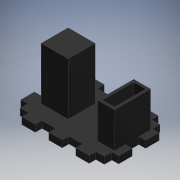
# Autodesk Inventor part: top
Saved by Autodesk Inventor 2019 (Build 230136000, 136)
## iProperties
Created: 2018-06-06
Part Number: top
Material: PBT Plastic Black
Document SubType Name: Modeling
Designer: stra92745
Density: 1.31 g/cm^3
Appearance: Smooth - White
Author: stra92745
Autodesk Inventor part; units mm, degrees
ref_plane "YZ Plane" through (0, 0, 0) normal (1, 0, 0) x (0, 1, 0)
ref_plane "XZ Plane" through (0, 0, 0) normal (0, 1, 0) x (-1, 0, 0)
ref_plane "XY Plane" through (0, 0, 0) normal (0, 0, 1) x (1, 0, 0)
sketch "Sketch1" plane through (0, 0, 0) normal (0, 1, 0) x (-1, 0, 0)
  line L0 (0, 0) -> (-58, 0)
  line L1 (-58, 0) -> (-58, -41)
  line L2 (-58, -41) -> (0, -41)
  line L3 (0, -41) -> (0, 0)
  line L4 (-45.5, -30) -> (-52.5, -30)
  line L5 (-52.5, -30) -> (-52.5, -11.5)
  line L6 (-52.5, -11.5) -> (-45.5, -11.5)
  line L7 (-45.5, -11.5) -> (-45.5, -30)
  dimension "d0" = 58
  dimension "d1" = 41
  dimension "d2" = 11.5
  dimension "d3" = 11
  dimension "d4" = 7
  dimension "d5" = 5.5
  constraints: 16 end point, 4 parallel, 2 horizontal, 2 perpendicular
  measures "d0" distance of L2.end L1.end
  measures "d1" distance of L1.end L0.end
  measures "d2" distance between parallel lines of L0 L6
  measures "d3" distance between parallel lines of L2 L4
  measures "d4" distance of L5.end L6.end
  measures "d5" distance between parallel lines of L1 L5
extrude "Extrusion1" add sketch "Sketch1" along normal blind 4
sketch "Sketch2" plane through (0, 4, 0) normal (0, 1, 0) x (1, 0, 0)
  line L0 (45.5, 11.5) -> (45.5, 30) projected
  line L1 (45.5, 30) -> (52.5, 30) projected
  line L2 (52.5, 30) -> (52.5, 11.5) projected
  line L3 (52.5, 11.5) -> (45.5, 11.5) projected
  line L4 (54, 31.5) -> (44, 31.5)
  line L5 (44, 31.5) -> (44, 10)
  line L6 (44, 10) -> (54, 10)
  line L7 (54, 10) -> (54, 31.5)
  point P0 (0, 0)
  dimension "d8" = 1.5
  constraints: 8 end point, 3 other
  measures "d8" distance between parallel lines of L1 L4
extrude "Extrusion2" add sketch "Sketch2" along normal blind 21
sketch "Sketch3" plane through (0, 4, 0) normal (0, 1, 0) x (1, 0, 0)
  line L0 (58, 41) -> (0, 41) construction
  line L1 (0, 41) -> (0, 0) construction
  line L2 (0, 0) -> (58, 0) construction
  line L3 (58, 0) -> (58, 41) construction
  line L4 (4, 37) -> (54, 37) construction
  line L5 (54, 37) -> (54, 4) construction
  line L6 (54, 4) -> (4, 4) construction
  line L7 (4, 4) -> (4, 37) construction
  line L8 (0, 20.5) -> (58, 20.5) construction
  line L9 (29, 0) -> (29, 41) construction
  line L10 (0, 16.5) -> (4, 16.5)
  line L11 (4, 16.5) -> (4, 20.5)
  line L12 (0, 16.5) -> (0, 20.5)
  line L13 (0, 8.5) -> (4, 8.5)
  line L14 (4, 8.5) -> (4, 4)
  line L15 (4, 4) -> (9, 4)
  line L16 (9, 4) -> (9, 0)
  line L17 (9, 0) -> (0, 0)
  line L18 (0, 0) -> (0, 8.5)
  line L19 (17, 4) -> (17, 0)
  line L20 (17, 0) -> (25, 0)
  line L21 (25, 0) -> (25, 4)
  line L22 (25, 4) -> (17, 4)
  line L23 (0, 24.5) -> (4, 24.5)
  line L24 (4, 24.5) -> (4, 20.5)
  line L25 (0, 24.5) -> (0, 20.5)
  line L26 (0, 32.5) -> (4, 32.5)
  line L27 (4, 32.5) -> (4, 37)
  line L28 (4, 37) -> (9, 37)
  line L29 (9, 37) -> (9, 41)
  line L30 (9, 41) -> (0, 41)
  line L31 (0, 41) -> (0, 32.5)
  line L32 (17, 37) -> (17, 41)
  line L33 (17, 41) -> (25, 41)
  line L34 (25, 41) -> (25, 37)
  line L35 (25, 37) -> (17, 37)
  line L36 (58, 41) -> (58, 0) construction
  line L37 (54, 4) -> (54, 37) construction
  line L38 (58, 16.5) -> (54, 16.5)
  line L39 (54, 16.5) -> (54, 20.5)
  line L40 (58, 16.5) -> (58, 20.5)
  line L41 (58, 8.5) -> (54, 8.5)
  line L42 (54, 8.5) -> (54, 4)
  line L43 (54, 4) -> (49, 4)
  line L44 (49, 4) -> (49, 0)
  line L45 (49, 0) -> (58, 0)
  line L46 (58, 0) -> (58, 8.5)
  line L47 (41, 4) -> (41, 0)
  line L48 (41, 0) -> (33, 0)
  line L49 (33, 0) -> (33, 4)
  line L50 (33, 4) -> (41, 4)
  line L51 (49, 37) -> (49, 41)
  line L52 (54, 24.5) -> (54, 20.5)
  line L53 (54, 32.5) -> (54, 37)
  line L54 (54, 37) -> (49, 37)
  line L55 (58, 24.5) -> (58, 20.5)
  line L56 (58, 24.5) -> (54, 24.5)
  line L57 (58, 32.5) -> (54, 32.5)
  line L58 (58, 41) -> (58, 32.5)
  line L59 (49, 41) -> (58, 41)
  line L60 (41, 37) -> (41, 41)
  line L61 (33, 37) -> (41, 37)
  line L62 (41, 41) -> (33, 41)
  line L63 (33, 41) -> (33, 37)
  dimension "d11" = 4
  dimension "d12" = 4
  dimension "d13" = 8
  dimension "d14" = 8
  dimension "d15" = 4
  dimension "d16" = 8
  constraints: 120 end point, 31 symmetric about line, 15 point on line, 7 perpendicular, 6 midpoint, 2 collinear, 1 vertical, 3 other
  measures "d11" distance between parallel lines of L0 L4
  measures "d12" distance of L10.end L11.end
  measures "d13" distance between parallel lines of L13 L10
  measures "d14" distance of L21.end L19.start
  measures "d15" distance between parallel lines of L9 L21
  measures "d16" distance between parallel lines of L16 L19
extrude "Extrusion3" cut sketch "Sketch3" against normal up to surface (4 mm away)
sketch "Sketch5" plane through (0, 4, 0) normal (0, 1, 0) x (1, 0, 0)
  line L0 (8, 28.5) -> (24, 28.5)
  line L1 (24, 28.5) -> (24, 12.5)
  line L2 (24, 12.5) -> (8, 12.5)
  line L3 (8, 12.5) -> (8, 28.5)
  line L4 (4, 24.5) -> (4, 16.5) construction
  line L5 (4, 16.5) -> (4, 24.5) construction
  line L6 (4, 20.5) -> (8, 20.5) construction
  point P0 (0, 0)
  dimension "d23" = 4
  dimension "d24" = 16
  dimension "d25" = 16
  constraints: 10 end point, 2 horizontal, 2 midpoint, 2 parallel, 1 perpendicular
  measures "d23" distance between parallel lines of L3 L4
  measures "d24" distance of L1.end L2.end
  measures "d25" distance of L0.end L1.end
extrude "Extrusion4" add sketch "Sketch5" along normal blind 31
body "Solid1"
